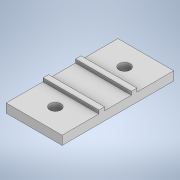
# Autodesk Inventor part: bodystandoff
Saved by Autodesk Inventor 2020.3 (Build 243373000, 373)
## iProperties
Created: 2021-06-21
Part Number: bodystandoff
Material: Generic
Document SubType Name: Modeling
Designer: 0x6f736f646f
Density: 1 g/cm^3
Appearance: Default
Author: 0x6f736f646f
Autodesk Inventor part; units mm, degrees
ref_plane "YZ Plane" through (0, 0, 0) normal (1, 0, 0) x (0, 1, 0)
ref_plane "XZ Plane" through (0, 0, 0) normal (0, 1, 0) x (-1, 0, 0)
ref_plane "XY Plane" through (0, 0, 0) normal (0, 0, 1) x (1, 0, 0)
sketch "Sketch1" plane through (0, 0, 0) normal (0, 1, 0) x (-1, 0, 0)
  line L0 (0, 0) -> (-50, 0)
  line L1 (-50, 0) -> (-50, -100)
  line L2 (-50, -100) -> (0, -100)
  line L3 (0, -100) -> (0, 0)
  circle A0 centre (-25, -18.9688) radius 5
  circle A1 centre (-25, -81.0312) radius 5
  line L4 (0, -37.9375) -> (-50, -37.9375)
  line L5 (0, -62.0625) -> (-50, -62.0625)
  line L6 (0, -32.9375) -> (-50, -32.9375)
  line L7 (0, -67.0625) -> (-50, -67.0625)
  dimension "d0" = 50
  dimension "d1" = 100
  dimension "d2" = 18.9688
  dimension "d3" = 18.9688
  dimension "d4" = 10
  dimension "d5" = 25
  dimension "d8" = 24.125
  dimension "d9" = 37.9375
  dimension "d10" = 5
  dimension "d11" = 5
  constraints: 16 end point, 4 parallel, 4 point on line, 3 perpendicular, 2 centre point, 1 equal radius, 1 horizontal, 1 vertical alignment
  measures "d0" distance of L2.end L1.end
  measures "d1" distance of L1.end L0.end
  measures "d2" distance from line of L2 A1.centre
  measures "d3" distance from line of L0 A0.centre
  measures "d4" diameter of A1
  measures "d5" distance from line of L3 A1.centre
  measures "d8" distance between parallel lines of L5 L4
  measures "d9" distance between parallel lines of L0 L4
  measures "d10" distance between parallel lines of L4 L6
  measures "d11" distance between parallel lines of L5 L7
extrude "Extrusion1" add sketch "Sketch1" along normal blind 7.9375
extrude "Extrusion2" add sketch "Sketch1" along normal blind 11 contours L3 L4 L1 L6 | L3 L7 L1 L5
body "Solid1"
